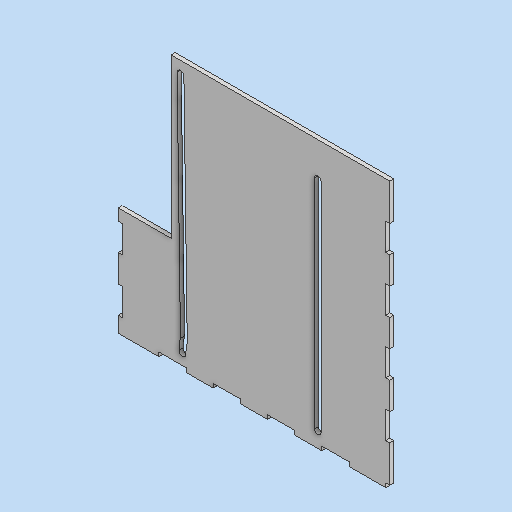
# Autodesk Inventor part: inside walls
Saved by Autodesk Inventor 2026 (Build 300175000, 175)
## iProperties
Created: 2026-02-03
Part Number: inside walls
Material: Generic
Document SubType Name: Modeling
Designer: mones
Density: 1 g/cm^3
Appearance: Default
Author: mones
Autodesk Inventor part; units mm, degrees
ref_plane "YZ Plane" through (0, 0, 0) normal (1, 0, 0) x (0, 1, 0)
ref_plane "XZ Plane" through (0, 0, 0) normal (0, 1, 0) x (-1, 0, 0)
ref_plane "XY Plane" through (0, 0, 0) normal (0, 0, 1) x (1, 0, 0)
sketch "Sketch1" plane through (0, 0, 0) normal (0, 0, 1) x (1, 0, 0)
  line L0 (6, 6) -> (200, 6)
  line L1 (200, 6) -> (200, 200)
  line L2 (200, 200) -> (42, 200)
  line L3 (6, 83) -> (6, 6)
  line L4 (6, 6) -> (56, 6)
  line L5 (200, 6) -> (150, 6)
  line L6 (200, 6) -> (200, 153)
  line L7 (150, 6) -> (142.5, 6)
  line L8 (200, 6) -> (200, 166)
  arc A0 (152.5, 174.3333) -> (147.5, 174.3333) centre (150, 174.3333) ccw
  line L9 (150, 6) -> (50, 6)
  arc A1 (47.8689, 14.6053) -> (52.8158, 14.5813) centre (50.3406, 14.23) ccw
  arc A2 (53.8259, 22.009) -> (52.8051, 13.8106) centre (86.918, 13.7258) ccw
  arc A3 (51.3944, 191.2047) -> (46.3962, 191.0801) centre (48.8946, 191.1682) ccw
  line L10 (53.8599, 22.4199) -> (51.3944, 191.2047)
  line L11 (48.8556, 22.7156) -> (46.3962, 191.0801)
  arc A4 (53.7373, 21.6465) -> (53.8589, 22.4929) centre (51.3599, 22.4199) ccw
  arc A5 (48.8556, 22.7156) -> (47.8689, 14.6053) centre (80.6169, 14.7362) ccw
  line L12 (52.8406, 14.23) -> (52.8088, 14.23)
  arc A6 (147.5, 14.23) -> (152.5, 14.23) centre (150, 14.23) ccw
  line L13 (147.5, 14.23) -> (147.5, 174.3333)
  line L14 (152.5, 14.23) -> (152.5, 174.3333)
  line L15 (42, 200) -> (42, 83)
  line L16 (42, 83) -> (6, 83)
  dimension "d1" = 194
  constraints: 35 end point, 20 point on circle, 7 centre point, 7 point on line, 4 tangent, 2 parallel, 2 perpendicular, 1 horizontal
  measures "d1" distance of L1.end L0.end
extrude "Extrusion1" add sketch "Sketch1" along normal blind 3
sketch "Sketch2" plane through (0, 0, 3) normal (0, 0, 1) x (1, 0, 0)
  line L0 (200, 6) -> (200, 200) projected
  line L1 (200, 200) -> (42, 200) projected
  line L2 (42, 200) -> (42, 83) projected
  line L3 (42, 83) -> (6, 83) projected
  line L4 (6, 83) -> (6, 6) projected
  line L5 (6, 6) -> (200, 6) projected
  line L6 (147.5, 14.23) -> (147.5, 174.3333) projected
  arc A0 (152.5, 174.3333) -> (147.5, 174.3333) centre (150, 174.3333) ccw projected
  line L7 (152.5, 174.3333) -> (152.5, 14.23) projected
  arc A1 (147.5, 14.23) -> (152.5, 14.23) centre (150, 14.23) ccw projected
  arc A2 (51.3944, 191.2047) -> (46.3962, 191.0801) centre (48.8946, 191.1682) ccw projected
  line L8 (51.3944, 191.2047) -> (53.8589, 22.4929) projected
  arc A3 (53.7373, 21.6465) -> (53.8589, 22.4929) centre (51.3599, 22.4199) ccw projected
  arc A4 (53.7373, 21.6465) -> (52.8158, 14.5813) centre (86.918, 13.7258) ccw projected
  arc A5 (47.8689, 14.6053) -> (52.8158, 14.5813) centre (50.3406, 14.23) ccw projected
  arc A6 (48.8556, 22.7156) -> (47.8689, 14.6053) centre (80.6169, 14.7362) ccw projected
  line L9 (48.8556, 22.7156) -> (46.3962, 191.0801) projected
  line L10 (6, 6) -> (33, 6)
  line L11 (33, 6) -> (53, 6)
  line L12 (53, 6) -> (73, 6)
  line L13 (73, 6) -> (93, 6)
  line L14 (93, 6) -> (113, 6)
  line L15 (113, 6) -> (133, 6)
  line L16 (133, 6) -> (153, 6)
  line L17 (153, 6) -> (173, 6)
  line L18 (6, 6) -> (6, 9)
  line L19 (33, 6) -> (33, 3)
  line L20 (173, 6) -> (173, 3)
  line L21 (53, 6) -> (53, 3)
  line L22 (93, 6) -> (93, 3)
  line L23 (73, 6) -> (73, 3)
  line L24 (133, 6) -> (133, 3)
  line L25 (113, 6) -> (113, 3)
  line L26 (153, 6) -> (153, 3)
  line L27 (6, 6) -> (6, 3)
  line L28 (6, 3) -> (33, 3)
  line L29 (173, 3) -> (200, 3)
  line L30 (200, 3) -> (200, 6.6126)
  line L31 (73, 3) -> (53, 3)
  line L32 (153, 3) -> (133, 3)
  line L33 (113, 3) -> (93, 3)
  point P0 (120.702, 9)
  point P1 (49.056, 9)
  constraints: 48 end point, 13 perpendicular, 4 point on line, 3 vertical, 2 parallel, 1 point on circle, 9 other
extrude "Extrusion2" add sketch "Sketch2" against normal blind 3 contours L30 L29 L20 L5 | L26 L32 L24 L5 | L25 L33 L22 L5 | L23 L31 L21 L5 | L5 L19 L28 L27
sketch "Sketch3" plane through (0, 0, 3) normal (0, 0, 1) x (1, 0, 0)
  line L0 (153, 6) -> (173, 6) projected
  line L1 (73, 6) -> (93, 6) projected
  line L2 (200, 3) -> (200, 200) projected
  line L3 (200, 200) -> (42, 200) projected
  line L4 (42, 200) -> (42, 83) projected
  line L5 (42, 83) -> (6, 83) projected
  line L6 (6, 83) -> (6, 3) projected
  line L7 (33, 6) -> (53, 6) projected
  line L8 (113, 6) -> (133, 6) projected
  line L9 (147.5, 14.23) -> (147.5, 174.3333) projected
  arc A0 (152.5, 174.3333) -> (147.5, 174.3333) centre (150, 174.3333) ccw projected
  line L10 (152.5, 174.3333) -> (152.5, 14.23) projected
  arc A1 (147.5, 14.23) -> (152.5, 14.23) centre (150, 14.23) ccw projected
  arc A2 (51.3944, 191.2047) -> (46.3962, 191.0801) centre (48.8946, 191.1682) ccw projected
  line L11 (51.3944, 191.2047) -> (53.8589, 22.4929) projected
  arc A3 (53.7373, 21.6465) -> (53.8589, 22.4929) centre (51.3599, 22.4199) ccw projected
  arc A4 (53.7373, 21.6465) -> (52.8158, 14.5813) centre (86.918, 13.7258) ccw projected
  arc A5 (47.8689, 14.6053) -> (52.8158, 14.5813) centre (50.3406, 14.23) ccw projected
  arc A6 (48.8556, 22.7156) -> (47.8689, 14.6053) centre (80.6169, 14.7362) ccw projected
  line L12 (48.8556, 22.7156) -> (46.3962, 191.0801) projected
  line L13 (6, 83) -> (6, 80)
  line L14 (6, 83) -> (3, 83)
  line L15 (3, 6) -> (3, 14.5)
  line L16 (3, 83) -> (3, 74.5)
  line L17 (3, 54.5) -> (3, 34.5)
  line L18 (3, 74.5) -> (6, 74.5)
  line L19 (3, 54.5) -> (6, 54.5)
  line L20 (3, 34.5) -> (6, 34.5)
  line L21 (3, 14.5) -> (6, 14.5)
  line L22 (3, 14.5) -> (3, 6)
  line L23 (3, 83) -> (3, 74.5)
  line L24 (3, 54.5) -> (3, 34.5)
  line L25 (3, 6) -> (3, 3)
  line L26 (3, 3) -> (6, 3)
  line L27 (6, 3) -> (6, 6)
  line L28 (6, 3) -> (33, 3) projected
  line L29 (33, 3) -> (33, 6) projected
  line L30 (53, 6) -> (53, 3) projected
  line L31 (53, 3) -> (73, 3) projected
  line L32 (73, 3) -> (73, 6) projected
  line L33 (93, 6) -> (93, 3) projected
  line L34 (93, 3) -> (113, 3) projected
  line L35 (113, 3) -> (113, 6) projected
  line L36 (133, 6) -> (133, 3) projected
  line L37 (133, 3) -> (153, 3) projected
  line L38 (153, 3) -> (153, 6) projected
  line L39 (173, 6) -> (173, 3) projected
  line L40 (173, 3) -> (200, 3) projected
  point P0 (6, 3)
  dimension "d43" = 3
  constraints: 30 end point, 5 perpendicular, 5 point on line, 1 horizontal, 1 parallel, 1 vertical
  measures "d43" distance of L5.end L14.end
extrude "Extrusion3" add sketch "Sketch3" against normal blind 3 contours L6 L18 L16 L14 | L6 L20 L17 L19 | L6 L26 L25 L15 L21
sketch "Sketch4" plane through (0, 0, 3) normal (0, 0, 1) x (1, 0, 0)
  line L0 (153, 6) -> (173, 6) projected
  line L1 (73, 6) -> (93, 6) projected
  line L2 (200, 200) -> (42, 200) projected
  line L3 (42, 200) -> (42, 83) projected
  line L4 (42, 83) -> (3, 83) projected
  line L5 (3, 83) -> (3, 74.5) projected
  line L6 (3, 74.5) -> (6, 74.5) projected
  line L7 (6, 74.5) -> (6, 54.5) projected
  line L8 (6, 54.5) -> (3, 54.5) projected
  line L9 (3, 54.5) -> (3, 34.5) projected
  line L10 (3, 34.5) -> (6, 34.5) projected
  line L11 (33, 6) -> (53, 6) projected
  line L12 (113, 6) -> (133, 6) projected
  line L13 (147.5, 14.23) -> (147.5, 174.3333) projected
  arc A0 (152.5, 174.3333) -> (147.5, 174.3333) centre (150, 174.3333) ccw projected
  line L14 (152.5, 174.3333) -> (152.5, 14.23) projected
  arc A1 (147.5, 14.23) -> (152.5, 14.23) centre (150, 14.23) ccw projected
  arc A2 (51.3944, 191.2047) -> (46.3962, 191.0801) centre (48.8946, 191.1682) ccw projected
  line L15 (51.3944, 191.2047) -> (53.8589, 22.4929) projected
  arc A3 (53.7373, 21.6465) -> (53.8589, 22.4929) centre (51.3599, 22.4199) ccw projected
  arc A4 (53.7373, 21.6465) -> (52.8158, 14.5813) centre (86.918, 13.7258) ccw projected
  arc A5 (47.8689, 14.6053) -> (52.8158, 14.5813) centre (50.3406, 14.23) ccw projected
  arc A6 (48.8556, 22.7156) -> (47.8689, 14.6053) centre (80.6169, 14.7362) ccw projected
  line L16 (48.8556, 22.7156) -> (46.3962, 191.0801) projected
  line L17 (200, 6) -> (203, 6)
  line L18 (200, 200) -> (203, 200)
  line L19 (200, 6) -> (200, 33)
  line L20 (200, 33) -> (200, 53)
  line L21 (200, 53) -> (200, 73)
  line L22 (200, 73) -> (200, 93)
  line L23 (200, 93) -> (200, 113)
  line L24 (200, 113) -> (200, 133)
  line L25 (200, 133) -> (200, 153)
  line L26 (200, 153) -> (200, 173)
  line L27 (200, 173) -> (200, 200)
  line L28 (200, 173) -> (203, 173)
  line L29 (200, 153) -> (203, 153)
  line L30 (200, 133) -> (203, 133)
  line L31 (200, 113) -> (203, 113)
  line L32 (200, 93) -> (203, 93)
  line L33 (200, 73) -> (203, 73)
  line L34 (200, 53) -> (203, 53)
  line L35 (200, 33) -> (203, 33)
  line L36 (203, 200) -> (203, 173)
  line L37 (203, 153) -> (203, 133)
  line L38 (203, 113) -> (203, 93)
  line L39 (203, 73) -> (203, 53)
  line L40 (203, 33) -> (203, 6)
  line L41 (200, 3) -> (200, 200) projected
  line L42 (6, 34.5) -> (6, 14.5) projected
  line L43 (3, 3) -> (33, 3) projected
  line L44 (33, 3) -> (33, 6) projected
  line L45 (53, 6) -> (53, 3) projected
  line L46 (53, 3) -> (73, 3) projected
  line L47 (73, 3) -> (73, 6) projected
  line L48 (93, 6) -> (93, 3) projected
  line L49 (93, 3) -> (113, 3) projected
  line L50 (113, 3) -> (113, 6) projected
  line L51 (133, 6) -> (133, 3) projected
  line L52 (133, 3) -> (153, 3) projected
  line L53 (153, 3) -> (153, 6) projected
  line L54 (173, 6) -> (173, 3) projected
  line L55 (173, 3) -> (200, 3) projected
  line L56 (6, 14.5) -> (3, 14.5) projected
  line L57 (3, 14.5) -> (3, 3) projected
  constraints: 48 end point, 30 perpendicular, 2 horizontal, 2 parallel
extrude "Extrusion4" add sketch "Sketch4" against normal blind 3 contours L19 L35 L40 L17 | L21 L33 L39 L34 | L23 L31 L38 L32 | L25 L29 L37 L30 | L27 L18 L36 L28
body "Solid1"
